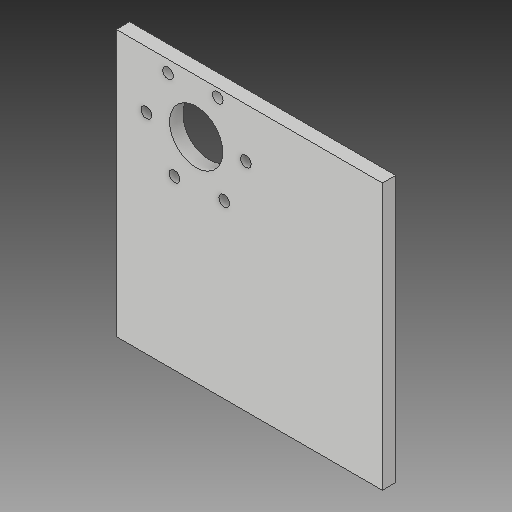
# Autodesk Inventor part: supportPlateForLinearActuator
Saved by Autodesk Inventor 2018.2 (Build 222227000, 227)
## iProperties
Created: 2018-01-09
Part Number: supportPlateForLinearActuator
Material: Generic
Document SubType Name: Modeling
Designer: steele
Density: 1 g/cm^3
Appearance: Default
Author: steele
Autodesk Inventor part; units mm, degrees
ref_plane "YZ Plane" through (0, 0, 0) normal (1, 0, 0) x (0, 1, 0)
ref_plane "XZ Plane" through (0, 0, 0) normal (0, 1, 0) x (-1, 0, 0)
ref_plane "XY Plane" through (0, 0, 0) normal (0, 0, 1) x (1, 0, 0)
sketch "Sketch1" plane through (0, 0, 0) normal (0, 0, 1) x (1, 0, 0)
  line L0 (-63.5, -63.5) -> (63.5, -63.5)
  line L1 (63.5, -63.5) -> (63.5, 63.5)
  line L2 (63.5, 63.5) -> (-63.5, 63.5)
  line L3 (-63.5, 63.5) -> (-63.5, -63.5)
  point P0 (0, 0)
  dimension "d19" = 63.5
  constraints: 8 end point, 2 parallel, 1 horizontal, 1 perpendicular
  measures "d19" distance from line of point (0, 0) L2
extrude "Extrusion1" add sketch "Sketch1" against normal blind 6.35
sketch "Sketch2" plane through (0, 0, 0) normal (0, 0, 1) x (1, 0, 0)
  circle A0 centre (-25.4, 38.1) radius 12.7
  line L0 (63.5, 63.5) -> (-63.5, 63.5) projected
  line L1 (-63.5, -63.5) -> (-63.5, 63.5) projected
  dimension "d4" = 25.4
  dimension "d20" = 25.4
  dimension "d23" = 38.1
  constraints: 1 centre point, 1 coincident
  measures "d4" diameter of A0
  measures "d20" distance from line of point (-25.4, 38.1) L0
  measures "d23" distance from line of point (-25.4, 38.1) L1
extrude "Extrusion2" cut sketch "Sketch2" against normal through all
sketch "Sketch3" plane through (0, 0, 0) normal (0, 0, 1) x (1, 0, 0)
  circle A0 centre (-25.4, 38.1) radius 23.8125 construction
  line L0 (63.5, 63.5) -> (-63.5, 63.5) projected
  line L1 (-63.5, 63.5) -> (-63.5, -63.5) projected
  point P0 (-15.0599, 59.5503)
  point P1 (-1.6534, 39.8703)
  point P2 (-11.9935, 18.42)
  point P3 (-35.7401, 16.6497)
  point P4 (-49.1466, 36.3297)
  point P5 (-38.8065, 57.78)
  dimension "d7" = 47.625
  dimension "d10" = 360
  dimension "d21" = 25.4
  dimension "d22" = 38.1
  constraints: 1 coincident, 10 other
  measures "d21" distance from line of point (-25.4, 38.1) L0
  measures "d22" distance from line of point (-25.4, 38.1) L1
hole "Hole1" at (-15.0599, 59.5503, 0) at (-1.6534, 39.8703, 0) at (-11.9935, 18.42, 0) at (-35.7401, 16.6497, 0) at (-49.1466, 36.3297, 0) at (-38.8065, 57.78, 0) direction (0, 0, -1) diameter 5.1054 end through all clearance for "Flat Head Machine Screw (82)" size "#10" standard "Ansi Unified Screw Threads"
body "Solid1"
